Link v19 (Autodesk Fusion 360 design; units mm, degrees)
Autodesk Fusion 360 part; units mm, degrees
sketch "Sketch1" plane through (0, 0, 0) normal (0, 1, 0) x (1, 0, 0)
  line L0 (0, 0) -> (50, 0)
  line L1 (50, 0) -> (50, -10)
  line L2 (50, -10) -> (0, -10)
  line L3 (0, -10) -> (0, 0)
  line L4 (0, -5) -> (50, -5) construction
  circle A0 centre (5, -5) radius 1.575
  dimension "d1" = 50
  dimension "d2" = 10
  dimension "d3" = 3.15
  dimension "d10" = 5
  constraint horizontal L0
  constraint vertical L1
  constraint horizontal L2
  constraint vertical L3
  constraint coincident L0.start L3.end
  constraint midpoint L3 L0.start
  constraint midpoint L1 L0.start
  constraint coincident L4 L0.start
  measures "d2" distance of L0.start L3.end L1
  measures "d3" diameter of A0
extrude "Extrude1" add sketch "Sketch1" along normal blind 3
sketch "Sketch2" plane through (0, 3, 0) normal (0, 1, 0) x (-1, 0, 0)
  circle A0 centre (-5, 5) radius 1.575
  line L0 (0, 10) -> (-50, 10)
  line L1 (-50, 10) -> (-50, 0)
  line L2 (-50, 0) -> (0, 0)
  line L3 (0, 0) -> (0, 10)
  line L4 (-43, 3) -> (-47, 3) construction
  line L5 (-47, 3) -> (-47, 7) construction
  line L6 (-47, 7) -> (-43, 7) construction
  line L7 (-43, 7) -> (-43, 3) construction
  line L8 (-43, 3) -> (-47, 7) construction
  line L9 (-47, 3) -> (-43, 7) construction
  circle A1 centre (-45, 5) radius 2
  dimension "d12" = 40
  dimension "d15" = 4
  constraint perpendicular L4 L5
  constraint parallel L4 L6
  constraint parallel L5 L7
  constraint horizontal L4
  constraint coincident L8 L2.end
  constraint coincident L9 L2.end
  constraint coincident L2.end L3.start
  measures "d15" diameter of A1
extrude "Extrude2" add sketch "Sketch2" along normal blind 10 contours A1
fillet "Fillet1" radius 5 4 edges at (0, 1.5, 0) (0, 1.5, 10) (50, 1.5, 0) (50, 1.5, 10)
sketch "Sketch3" plane through (0, 13, 0) normal (0, 1, 0) x (-1, 0, 0)
  circle A0 centre (-45, 5) radius 2
  circle A1 centre (-45, 5) radius 1
  dimension "d16" = 2
  constraint concentric A0 A1
  measures "d16" diameter of A1
extrude "Extrude3" cut sketch "Sketch3" against normal through all contours A1
